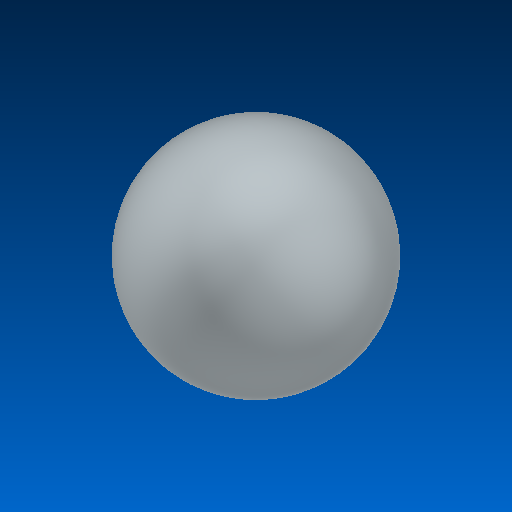
# Autodesk Inventor part: 1- HUDSON-8-31-TDR HAND PUMP PISTON
Saved by Autodesk Inventor 2025.2 (Build 292293000, 293)
## iProperties
Created: 2024-11-02
Part Number: 1- HUDSON-8-31-TDR HAND PUMP PISTON
Material: Genérico
Document SubType Name: Modeling
Designer: brene
Density: 1 g/cm^3
Appearance: Zinc
Author: brene
Autodesk Inventor part; units mm, degrees
ref_plane "YZ Plane" through (0, 0, 0) normal (1, 0, 0) x (0, 1, 0)
ref_plane "XZ Plane" through (0, 0, 0) normal (0, 1, 0) x (-1, 0, 0)
ref_plane "XY Plane" through (0, 0, 0) normal (0, 0, 1) x (1, 0, 0)
sketch "Boceto1" plane through (0, 0, 0) normal (0, 0, 1) x (1, 0, 0)
  line L0 (0, 219.3887) -> (0, -219.3887)
  arc A0 (0, -3) -> (0, 3) centre (0, 0) ccw
  dimension "d3" = 219.3887
  dimension "d6" = 6
  constraints: 2 coincident, 2 end point, 2 point on circle, 2 point on line, 1 centre point, 1 midpoint, 1 vertical
  measures "d3" distance of L0.start point (0, 0)
  measures "d6" diameter of A0
revolve "Revolución1" add sketch "Boceto1" angle 360 about axis through (0, 219.3887, 0) along (0, -1, 0)
